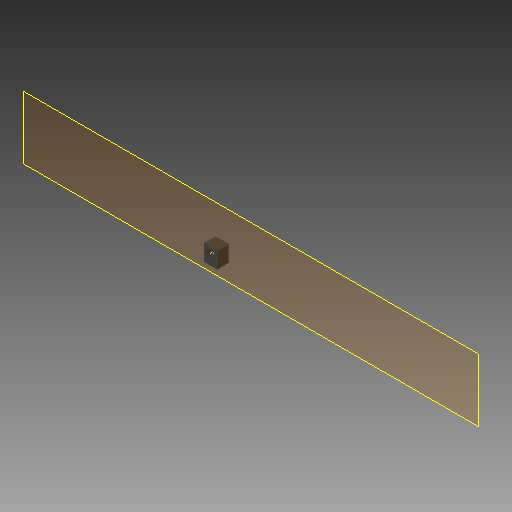
# Autodesk Inventor part: AUDIO DC12
Saved by Autodesk Inventor 2017 SP1 (Build 210196100, 196)
## iProperties
Created: 2021-02-22
Part Number: AUDIO DC12
Material: Tworzywo sztuczne, nieprzezroczyste czarne
Document SubType Name: Modeling
Designer: Napoleon
Mass: 0.562225 g
Surface Area: 7.06939 cm^2
Volume: 0.590572 cm^3
Density: 0.952 g/cm^3
Appearance: Gładkie - czarne
Author: Napoleon
Autodesk Inventor part; units mm, degrees
ref_plane "YZ Plane" through (0, 0, 0) normal (1, 0, 0) x (0, 1, 0)
ref_plane "XZ Plane" through (0, 0, 0) normal (0, 1, 0) x (-1, 0, 0)
ref_plane "XY Plane" through (0, 0, 0) normal (0, 0, 1) x (1, 0, 0)
ref_plane "Płaszczyzna konstrukcyjna1" through (0, 0, 0) normal (0, 0, 1) x (1, 0, 0)
sketch "Szkic1" plane through (0, 0, 0) normal (0, 0, 1) x (1, 0, 0)
  line L0 (-32.2, -16.4467) -> (-32.2, -4.9467) projected
  line L1 (-32.2, -4.9467) -> (-22.7, -4.9467) projected
  line L2 (-22.7, -4.9467) -> (-22.7, -16.4467) projected
  line L3 (-22.7, -16.4467) -> (-32.2, -16.4467) projected
  line L4 (-31.95, -5.1967) -> (-22.95, -5.1967)
  line L5 (-22.95, -5.1967) -> (-22.95, -16.1967)
  line L6 (-22.95, -16.1967) -> (-31.95, -16.1967)
  line L7 (-31.95, -16.1967) -> (-31.95, -5.1967)
  circle A0 centre (-27.45, -9.3217) radius 3.125
  point P0 (0, 0)
  dimension "d0" = 9
  dimension "d1" = 11
  dimension "d2" = 6.25
  constraints: 8 end point, 2 parallel, 1 centre point, 1 horizontal, 1 perpendicular
  measures "d0" distance of L5.end L6.end
  measures "d1" distance of L4.end L5.end
  measures "d2" diameter of A0
extrude "Wyciągnięcie proste1" add sketch "Szkic1" against normal blind 6.5 and the other way blind 0.5 contours L4 L5 L6 L7
chamfer "Faza1" distance 0.25 angle 45 5 edges at (-27.45, -5.1967, 0.5) (-22.95, -10.6967, 0.5) (-31.95, -10.6967, 0.5) (-27.45, -16.1967, 0.5) (-30.575, -9.3217, 0.5)
sketch "Szkic2" plane through (0, 0, -6.5) normal (0, 0, -1) x (-1, 0, 0)
  circle A0 centre (27.45, -9.3217) radius 1
  circle A1 centre (27.45, -9.3217) radius 0.5
  point P0 (0, 0)
  dimension "d11" = 2
  dimension "d12" = 1
  constraints: 2 centre point, 2 coincident
  measures "d11" diameter of A0
  measures "d12" diameter of A1
extrude "Wyciągnięcie proste2" add sketch "Szkic2" against normal blind 6.5
fillet "Zaokrąglenie1" radius 0.25 1 edges at (-26.45, -9.3217, 0)
fillet "Zaokrąglenie2" radius 0.25 1 edges at (-26.95, -9.3217, 0)
sketch "Szkic3" plane through (0, 0, -6.5) normal (0, 0, -1) x (-1, 0, 0)
  line L0 (31.95, -5.1967) -> (22.95, -5.1967) projected
  line L1 (22.95, -5.1967) -> (22.95, -16.1967) projected
  line L2 (22.95, -16.1967) -> (31.95, -16.1967) projected
  line L3 (31.95, -16.1967) -> (31.95, -5.1967) projected
  point P0 (0, 0)
extrude "Wyciągnięcie proste3" add sketch "Szkic3" along normal blind 1
